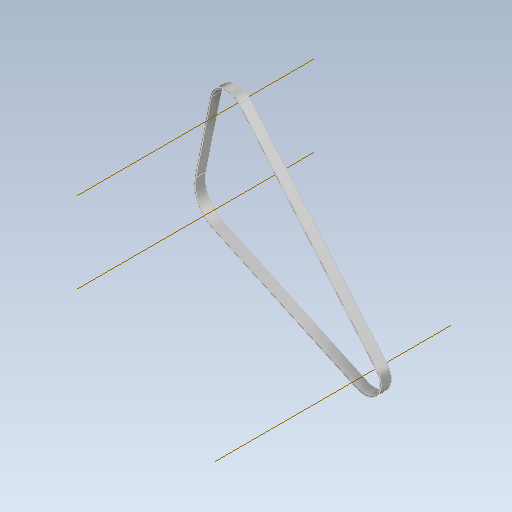
# Autodesk Inventor part: Зубчатый ремень
Saved by Autodesk Inventor 2021 (Build 250183000, 183)
## iProperties
Created: 2021-06-15
Part Number: Зубчатый ремень
Material: Rubber
Document SubType Name: Modeling
Designer: panda
Density: 1 g/cm^3
Appearance: Rubber - Black - Version 1.1
CustomPartVersion: 1
Author: panda
Autodesk Inventor part; units mm, degrees
sketch "Эскизная траектория" plane through (0, 0, 0) normal (0, 0, 1) x (1, 0, 0)
  arc A0 (-38.6417, 7.7676) -> (-16.4895, -35.7997) centre (0, 0) ccw
  arc A1 (15.0158, 112.7634) -> (-19.3209, 103.8838) centre (0, 100) ccw
  arc A2 (161.7553, -117.8998) -> (185.0158, -87.2366) centre (170, -100) ccw
  line L0 (161.7553, -117.8998) -> (-16.4895, -35.7997)
  line L1 (-38.6417, 7.7676) -> (-19.3209, 103.8838)
  line L2 (15.0158, 112.7634) -> (185.0158, -87.2366)
  constraints: 6 end point, 6 point on circle, 3 centre point
ref_plane "Плоскость сечения" through (-16.4895, -35.7997, 0) normal (0.9083, -0.4184, 0) x (0, 0, 1)
ref_plane "РабПлоскость2" through (0, 0, 0) normal (-1, 0, 0) x (0, 0, 1)
ref_plane "РабПлоскость3" through (0, 100, 0) normal (-0.3756, -0.9268, 0) x (0, 0, 1)
ref_plane "РабПлоскость4" through (170, -100, 0) normal (-0.5724, 0.8199, 0) x (0, 0, 1)
sketch "Сечение" plane through (-16.4895, -35.7997, 0) normal (0.9083, -0.4184, 0) x (0, 0, 1)
  line L0 (-6.35, 1.27) -> (6.35, 1.27)
  line L1 (6.35, 1.27) -> (6.35, -0.381)
  line L2 (6.35, -0.381) -> (-6.35, -0.381)
  line L3 (-6.35, -0.381) -> (-6.35, 1.27)
  line L4 (-6.35, 0) -> (6.35, 0) construction
  point P0 (0, 0)
  point P1 (0, 0)
  dimension "d0" = 12.7
  dimension "d4" = 0.381
  dimension "d5" = 1.27
  constraints: 10 end point, 2 parallel, 2 point on line, 1 coincident, 1 horizontal, 1 midpoint, 1 perpendicular, 1 other
  measures "d0" distance between parallel lines of L1 L3
  measures "d4" distance between parallel lines of L2 L4
  measures "d5" distance between parallel lines of L4 L0
sweep "Ремень" add profiles "Сечение" path "Эскизная траектория"
equation "\"d0\" = da_B"
equation "\"d4\" = da_a"
equation "\"d5\" = da_a2"
equation "\"da_B\" = 12.7"
equation "\"da_pb\" = 9.525"
equation "\"da_L\" = 706.95496"
equation "\"da_a\" = 0.381"
equation "\"da_S\" = 4.6482"
equation "\"da_Beta\" = 20deg"
equation "\"da_Ht\" = 1.905"
equation "\"da_H\" = 3.556"
equation "\"da_a2\" = 1.27"
body "Solid1"
